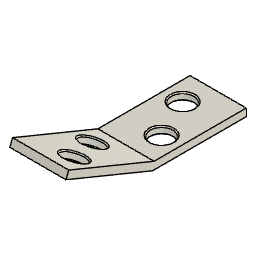
name_sign_bottom_bracket (Autodesk Fusion 360 design; units mm, degrees)
Autodesk Fusion 360 part; units mm, degrees
sketch "Sketch1" plane through (0, 0, 0) normal (1, 0, 0) x (0, 1, 0)
  line L0 (25, 0) -> (0, 0)
  line L1 (0, 0) -> (-23.1302, 9.4864)
  line L2 (-23.1302, 9.4864) -> (-22.3713, 11.3368)
  line L3 (-22.3713, 11.3368) -> (0.3942, 2)
  line L4 (0.3942, 2) -> (25, 2)
  line L5 (25, 2) -> (25, 0)
  dimension "d1" = 157.7
  dimension "d2" = 2
  dimension "d3" = 2
  dimension "d4" = 25
  dimension "d5" = 25
  constraint coincident L0.end L1.start
  constraint horizontal L0
  constraint perpendicular L1 L2
  constraint perpendicular L2 L3
  constraint horizontal L4
  constraint perpendicular L0 L5
  measures "d1" angle of L3 L4
  measures "d2" distance of L0.start L4.end
  measures "d3" distance of L1.end L2.end
  measures "d4" distance of L0.end L1.end
  measures "d5" distance of L0.start L0.end
extrude "Extrude1" add sketch "Sketch1" against normal blind 15
sketch "Sketch2" plane through (0, 0, 2) normal (0, 0, 1) x (-1, 0, 0)
  line L0 (0, -0.3942) -> (0, -25)
  line L1 (0, -25) -> (15, -25)
  line L2 (15, -25) -> (15, -0.3942)
  line L3 (15, -0.3942) -> (0, -0.3942)
  circle A0 centre (5, -7.3942) radius 3
  circle A1 centre (10, -18) radius 3
  dimension "d8" = 6
  dimension "d9" = 6
  dimension "d10" = 5
  dimension "d11" = 5
  dimension "d12" = 7
  dimension "d14" = 7
  measures "d8" diameter of A0
  measures "d9" diameter of A1
  measures "d10" distance of L2 A1.centre
  measures "d11" distance of L0 A0.centre
  measures "d12" distance of L1 A1.centre
  measures "d14" distance of L3 A0.centre
sketch "Sketch3" plane through (0, 0.7589, 1.8504) normal (0, 0.379456, 0.92521) x (-1, 0, 0)
  line L0 (0, 25) -> (0, 0.3942)
  line L1 (0, 0.3942) -> (15, 0.3942)
  line L2 (15, 0.3942) -> (15, 25)
  line L3 (15, 25) -> (0, 25)
  circle A0 centre (10, 7.3942) radius 3
  circle A1 centre (5, 18) radius 3
  dimension "d15" = 6
  dimension "d16" = 6
  dimension "d17" = 5
  dimension "d18" = 5
  dimension "d19" = 7
  dimension "d20" = 7
  measures "d15" diameter of A0
  measures "d16" diameter of A1
  measures "d17" distance of L0 A1.centre
  measures "d18" distance of L2 A0.centre
  measures "d19" distance of L3 A1.centre
  measures "d20" distance of L1 A0.centre
extrude "Extrude2" cut sketch "Sketch3" against normal blind 2 contours A0 | A1
extrude "Extrude3" cut sketch "Sketch2" against normal blind 2 contours A0 | A1
fillet "Fillet1" radius 0.3 8 edges at (-2.203, -16.8986, 9.0923) (-7.203, -7.086, 5.0678) (-2.203, 6.3094, 2) (-7.203, 16.9152, 2) (-2.203, -15.6501, 6.4186) (-7.203, -5.8375, 2.3941) (-2.203, 8.479, 0) (-7.203, 19.0848, 0)
named bodies: "Name Sign Bottom and Unsorted Smarties Top Connector"
